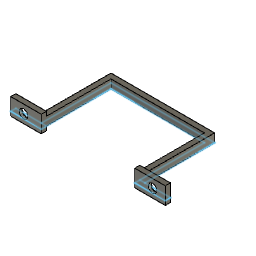
Extension Cord bracket v3 (Autodesk Fusion 360 design; units mm, degrees)
Autodesk Fusion 360 part; units mm, degrees
sketch "Sketch1" plane through (0, 0, 0) normal (0, 0, 1) x (1, 0, 0)
  line L0 (36.0554, 51.2556) -> (91.0554, 51.2556)
  line L1 (91.0554, 51.2556) -> (91.0554, 10.2556)
  line L2 (36.0554, 10.2556) -> (36.0554, 51.2556)
  line L3 (33.0554, 13.2556) -> (33.0554, 54.2556)
  line L4 (33.0554, 54.2556) -> (94.0554, 54.2556)
  line L5 (36.0554, 10.2556) -> (18.0554, 10.2556)
  line L6 (18.0554, 10.2556) -> (18.0554, 13.2556)
  line L7 (18.0554, 13.2556) -> (33.0554, 13.2556)
  line L8 (91.0554, 10.2556) -> (109.0554, 10.2556)
  line L9 (109.0554, 10.2556) -> (109.0554, 13.2556)
  line L10 (109.0554, 13.2556) -> (94.0554, 13.2556)
  line L11 (94.0554, 54.2556) -> (94.0554, 13.2556)
  line L12 (33.0554, 13.2556) -> (36.0554, 13.2556)
  line L13 (94.0554, 13.2556) -> (91.0554, 13.2556)
  dimension "d1" = 55
  dimension "d2" = 41
  dimension "d4" = 18
  dimension "d5" = 3
  dimension "d6" = 18
  dimension "d7" = 3
  constraint horizontal L0
  constraint vertical L1
  constraint vertical L2
  constraint perpendicular L3 L5
  constraint perpendicular L5 L6
  constraint perpendicular L3 L7
  constraint parallel L2 L3
  constraint parallel L0 L4
  constraint parallel L1 L11
  constraint perpendicular L1 L8
  constraint perpendicular L8 L9
  constraint perpendicular L10 L11
  constraint coincident L2 L12.end
  constraint perpendicular L2 L12
  constraint coincident L1 L13.end
  constraint perpendicular L1 L13
  measures "d1" distance of L0.start L0.end
  measures "d2" distance of L0.start L2.start
  measures "d4" distance of L2.start L5.end
  measures "d5" distance of L5.end L6.end
  measures "d6" distance of L1.end L8.end
  measures "d7" distance of L8.end L9.end
extrude "Extrude3" add sketch "Sketch1" along normal blind 7.5 contours L2 L5 L6 L7 L12 | L1 L8 L9 L10 L13 makes body 1 at (30.0554, 10.2556, 2.5) makes body 2 at (103.0554, 13.2556, 2.5)
extrude "Extrude2" add sketch "Sketch1" along normal blind 5 separate body contours L0 L1 L2 L3 L4 L11 L12 L13 makes body 3
extrude "Extrude4" add sketch "Sketch1" against normal blind 2.5 contours L2 L5 L6 L7 L12 | L1 L8 L9 L10 L13 bodies 1 2 3
hole "Hole1" at (25.5554, 13.2556, 2.5) direction (0, -1, 0) diameter 5 depth 10 tip angle 118 countersink diameter 8 countersink angle 90 bodies 1
ref_plane "WorkPlane1" through (63.5554, 33.7556, 2.5) normal (-1, 0, 0) x (0, -1, 0)
mirror "Mirror1" about plane through (63.5554, 33.7556, 2.5) normal (-1, 0, 0) of "Hole1"
